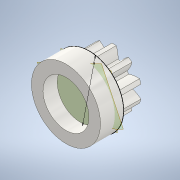
# Autodesk Inventor part: Spur Gear2
Saved by Autodesk Inventor 2022 (Build 260153070, 153G)
## iProperties
CustomPartVersion: 1
Created: 2021-10-29
Part Number: Spur Gear2
Material: Steel
Document SubType Name: Modeling
Designer: a laptop
Categories: <?xml version="1.0" encoding="UTF-16"?> <MemberInstance><Categories><FamilyTemplate><FamilyTemplateParameter ValueType="xs:double" Id="1" ObjectReferenceKey="da_z" ObjectType="kUserParameterObject"/><FamilyTemplateParameter ValueType="xs:double" Id="2" ObjectReferenceKey="da_b" ObjectType="kUserParameterObject"/><FamilyTemplateParameter ValueType="xs:double" Id="3" ObjectReferenceKey="da_beta" ObjectType="kUserParameterObject"/><FamilyTemplateParameter ValueType="xs:double" Id="4" ObjectReferenceKey="da_da" ObjectType="kUserParameterObject"/><FamilyTemplateParameter ValueType="xs:double" Id="5" ObjectReferenceKey="da_aw" ObjectType="kUserParameterObject"/><FamilyTemplateParameter ValueType="xs:string" Id="6" ObjectReferenceKey="EAIAABAAAACIAQAAAAAAAIAAAAAAAAAA" ObjectType="83910656" SubObjectId="SurfaceGeometry"/></FamilyTemplate><ParamToTemplateMap><ParamToTemplate CategoryParameter="//CategoryParameter[@InternalName='046C89C9-8512-4d59-83FE-43B91F4F132A']" TemplateParameter="1"/><ParamToTemplate CategoryParameter="//CategoryParameter[@InternalName='2552DF32-E462-4b46-AEBF-C6C7768E72AC']" TemplateParameter="2"/><ParamToTemplate CategoryParameter="//CategoryParameter[@InternalName='C9EE641D-15FC-4fae-A226-E94C4372FDD7']" TemplateParameter="3"/><ParamToTemplate><ParamToTemplate CategoryParameter="//CategoryParameter[@InternalName='00B6519A-459B-49c7-AD84-2E56D39A5744']" ConstantValue="0.000000"/></ParamToTemplate><ParamToTemplate><ParamToTemplate CategoryParameter="//CategoryParameter[@InternalName='04B31F0E-C7A6-4894-AA32-9629BEFACF47']" ConstantValue="1.000000"/></ParamToTemplate><ParamToTemplate><ParamToTemplate CategoryParameter="//CategoryParameter[@InternalName='43CBEC2E-7847-49e7-A936-2F7889FCB2D9']" ConstantValue="0.250000"/></ParamToTemplate><ParamToTemplate><ParamToTemplate CategoryParameter="//CategoryParameter[@InternalName='B1EFC894-105D-4ebd-86BF-FA20ED196853']" ConstantValue="0.302500"/></ParamToTemplate><ParamToTemplate><ParamToTemplate CategoryParameter="//CategoryParameter[@InternalName='51175063-3D10-4879-93E8-6246FE8B403D']" ConstantValue="2060000000.000000"/></ParamToTemplate><ParamToTemplate><ParamToTemplate CategoryParameter="//CategoryParameter[@InternalName='A3A52E27-4454-46a9-B0BD-C932399B70AF']" ConstantValue="0.300000"/></ParamToTemplate><ParamToTemplate><ParamToTemplate CategoryParameter="//CategoryParameter[@InternalName='91B76062-C214-41d9-B1B9-14D2AB99603D']" ConstantValue="0.060000"/></ParamToTemplate><ParamToTemplate><ParamToTemplate CategoryParameter="//CategoryParameter[@InternalName='374E806E-8B8A-4dda-A9AA-1039D6500AD2']" ConstantValue="16.666667"/></ParamToTemplate><ParamToTemplate><ParamToTemplate CategoryParameter="//CategoryParameter[@InternalName='2D373A89-B862-43d6-8D0B-0CBF12AB9F6C']" ConstantValue="0.349066"/></ParamToTemplate><ParamToTemplate CategoryParameter="//CategoryParameter[@InternalName='37777632-D6A2-4fac-9D53-DB8ACD95C989']" TemplateParameter="4"/><ParamToTemplate CategoryParameter="//CategoryParameter[@InternalName='FD1017F1-B727-4f7e-9707-0F86F1FF9423']" TemplateParameter="5"/><ParamToTemplate><ParamToTemplate CategoryParameter="//CategoryParameter[@InternalName='9E1B4470-B2D3-4ff1-B813-535BB4CDF51A']" ConstantValue="3520000.000000"/></ParamToTemplate><ParamToTemplate><ParamToTemplate CategoryParameter="//CategoryParameter[@InternalName='F8452263-BFF6-458c-9FB1-07C4B99E95CD']" ConstantValue="11400000.000000"/></ParamToTemplate><ParamToTemplate><ParamToTemplate CategoryParameter="//CategoryParameter[@InternalName='3E3BB259-FD49-497f-8171-6EBC954A3479']" ConstantValue="2.000000"/></ParamToTemplate><ParamToTemplate CategoryParameter="//CategoryParameter[@InternalName='27C3BAF2-7550-4e4b-AE2C-0DB134B7D9B7']" TemplateParameter="6"/></ParamToTemplateMap><Category DisplayName="Gear" InternalName="DC85795E-93AB-48d5-8EEE-5A27447B64BD" Mnemonic="Gear"><CategoryParameter DisplayName="z" InternalName="046C89C9-8512-4d59-83FE-43B91F4F132A" Mnemonic="z"/><CategoryParameter DisplayName="b" InternalName="2552DF32-E462-4b46-AEBF-C6C7768E72AC" Mnemonic="b"/><CategoryParameter DisplayName="||b|" InternalName="C9EE641D-15FC-4fae-A226-E94C4372FDD7" Mnemonic="beta"/><CategoryParameter DisplayName="x" InternalName="00B6519A-459B-49c7-AD84-2E56D39A5744" Mnemonic="x"/><CategoryParameter DisplayName="a*" InternalName="04B31F0E-C7A6-4894-AA32-9629BEFACF47" Mnemonic="a"/><CategoryParameter DisplayName="c*" InternalName="43CBEC2E-7847-49e7-A936-2F7889FCB2D9" Mnemonic="c"/><CategoryParameter DisplayName="r|.f|*" InternalName="B1EFC894-105D-4ebd-86BF-FA20ED196853" Mnemonic="rf"/><CategoryParameter DisplayName="E" InternalName="51175063-3D10-4879-93E8-6246FE8B403D" Mnemonic="E"/><CategoryParameter DisplayName="||m|" InternalName="A3A52E27-4454-46a9-B0BD-C932399B70AF" Mnemonic="mi"/><Category DisplayName="SpurGear" InternalName="26C5A22E-A91E-4dfd-A3B3-23CCAFAE1764" Mnemonic="SpurGear"><CategoryParameter DisplayName="m" InternalName="91B76062-C214-41d9-B1B9-14D2AB99603D" Mnemonic="m"/><CategoryParameter DisplayName="P" InternalName="374E806E-8B8A-4dda-A9AA-1039D6500AD2" Mnemonic="PP"/><CategoryParameter DisplayName="||a|" InternalName="2D373A89-B862-43d6-8D0B-0CBF12AB9F6C" Mnemonic="alpha"/><CategoryParameter DisplayName="d|.a|" InternalName="37777632-D6A2-4fac-9D53-DB8ACD95C989" Mnemonic="da"/><CategoryParameter DisplayName="a|.w|" InternalName="FD1017F1-B727-4f7e-9707-0F86F1FF9423" Mnemonic="aw"/><CategoryParameter DisplayName="||s||.Flim|" InternalName="9E1B4470-B2D3-4ff1-B813-535BB4CDF51A" Mnemonic="sFlim"/><CategoryParameter DisplayName="||s||.Hlim|" InternalName="F8452263-BFF6-458c-9FB1-07C4B99E95CD" Mnemonic="sHlim"/><CategoryParameter DisplayName="type" InternalName="3E3BB259-FD49-497f-8171-6EBC954A3479" Mnemonic="type"/><CategoryParameter DisplayName="PitchDiameter" InternalName="27C3BAF2-7550-4e4b-AE2C-0DB134B7D9B7" Mnemonic="IDS_PITCHDIAM"/></Category></Category></Categories></MemberInstance>
Density: 1 g/cm^3
Appearance: Steel
Author: a laptop
Autodesk Inventor part; units mm, degrees
ref_plane "YZ Plane" through (0, 0, 0) normal (1, 0, 0) x (0, 1, 0)
ref_plane "XZ Plane" through (0, 0, 0) normal (0, 1, 0) x (-1, 0, 0)
ref_plane "XY Plane" through (0, 0, 0) normal (0, 0, 1) x (1, 0, 0)
sketch "Sketch1" plane through (0, 0, 0) normal (0, 0, 1) x (1, 0, 0)
  circle A0 centre (0, 0) radius 3.6
  dimension "d0" = 7.2
  constraints: 1 centre point
  measures "d0" diameter of A0
extrude "Extrusion1" add sketch "Sketch1" along normal mid plane 3
ref_plane "Work Plane2" through (0, 0, 0) normal (0, 0, 1) x (1, 0, 0)
sketch "Sketch2" plane through (0, 0, -1.5) normal (0, 0, -1) x (-1, 0, 0)
  circle A0 centre (0, 0) radius 3.6 projected
  circle A1 centre (0, 0) radius 3
  dimension "d3" = 6
  constraints: 1 centre point, 1 coincident
  measures "d3" diameter of A1
surface extrude "Pitch Diameter" sketch "Sketch2" against normal through all shown no curves A1
ref_plane "Work Plane8" through (0, 0, 0) normal (0.9510565, 0.309017, 0) x (0, 0, 1)
ref_plane "Work Plane9" through (0, 0, 0) normal (1, 0, 0) x (0, 1, 0)
spur gear teeth "Spur Gear" teeth 10 pitch diameter 6 tip diameter 7.2 root diameter 4.5 face width 3 start plane through (0, 0, -1.5) normal (0, 0, -1) x (-1, 0, 0)
ref_plane "Work Plane12" through (0, 0, 2.9078) normal (0, 0, -1) x (-0.9035673, -0.4284463, 0)
ref_plane "Work Plane14" through (0, 0, 1.7684) normal (0, 0, -1) x (0.1129829, -0.9935969, 0)
sketch "Sketch6" plane through (0, 0, 1.7684) normal (0, 0, -1) x (0.1129829, -0.9935969, 0)
  arc A0 (-3.5978, -0.1248) -> (-3.534, -0.6861) centre (0, 0) ccw projected
  arc A1 (-0.9513, -2.039) -> (-0.9931, -3.4603) centre (2.2346, -2.8438) ccw projected
  arc A2 (-3.2624, 1.5221) -> (-2.1627, 0.6207) centre (-0.6786, 3.5524) ccw projected
  arc A3 (-3.5978, -0.1248) -> (-3.534, -0.6861) centre (0, 0) ccw projected
  arc A4 (-2.1627, 0.6207) -> (-2.2332, 0.2747) centre (0, 0) ccw projected
  arc A5 (-3.534, -0.6861) -> (-2.1145, -0.7691) centre (-2.6371, 2.4751) ccw projected
  arc A6 (-1.9681, -1.0904) -> (-2.8373, -2.2158) centre (0.1363, -3.6141) ccw projected
  arc A7 (-2.2332, 0.2747) -> (-3.5978, -0.1248) centre (-2.0141, -3.004) ccw projected
  arc A8 (-3.5978, -0.1248) -> (-3.534, -0.6861) centre (0, 0) ccw projected
  arc A9 (-2.1145, -0.7691) -> (-1.9681, -1.0904) centre (0, 0) ccw projected
  arc A10 (-1.2586, -1.8651) -> (-0.9513, -2.039) centre (0, 0) ccw projected
  arc A11 (-2.8373, -2.2158) -> (-2.4558, -2.6323) centre (0, 0) ccw projected
  arc A12 (-0.9931, -3.4603) -> (-0.4395, -3.5731) centre (0, 0) ccw projected
  arc A13 (-0.4395, -3.5731) -> (0.078, -2.2486) centre (-3.1689, -1.7432) ccw projected
  arc A14 (0.078, -2.2486) -> (0.4288, -2.2088) centre (0, 0) ccw projected
  arc A15 (0.4288, -2.2088) -> (1.2305, -3.3832) centre (3.4793, -0.9872) ccw projected
  arc A16 (1.2305, -3.3832) -> (1.7446, -3.149) centre (0, 0) ccw projected
  arc A17 (1.7446, -3.149) -> (1.3848, -1.7733) centre (-1.539, -3.2729) ccw projected
  arc A18 (1.3848, -1.7733) -> (1.6452, -1.5349) centre (0, 0) ccw projected
  arc A19 (1.6452, -1.5349) -> (2.9841, -2.0138) centre (3.3951, 1.2464) ccw projected
  arc A20 (2.9841, -2.0138) -> (3.2624, -1.5221) centre (0, 0) ccw projected
  arc A21 (3.2624, -1.5221) -> (2.1627, -0.6207) centre (0.6786, -3.5524) ccw projected
  arc A22 (2.1627, -0.6207) -> (2.2332, -0.2747) centre (0, 0) ccw projected
  arc A23 (2.2332, -0.2747) -> (3.5978, 0.1248) centre (2.0141, 3.004) ccw projected
  arc A24 (3.534, 0.6861) -> (2.1145, 0.7691) centre (2.6371, -2.4751) ccw projected
  arc A25 (-3.5978, -0.1248) -> (-3.534, -0.6861) centre (0, 0) ccw projected
  arc A26 (2.1145, 0.7691) -> (1.9681, 1.0904) centre (0, 0) ccw projected
  arc A27 (1.9681, 1.0904) -> (2.8373, 2.2158) centre (-0.1363, 3.6141) ccw projected
  arc A28 (-3.5978, -0.1248) -> (-3.534, -0.6861) centre (0, 0) ccw projected
  arc A29 (2.4558, 2.6323) -> (1.2586, 1.8651) centre (3.5883, -0.4523) ccw projected
  arc A30 (1.2586, 1.8651) -> (0.9513, 2.039) centre (0, 0) ccw projected
  arc A31 (0.9513, 2.039) -> (0.9931, 3.4603) centre (-2.2346, 2.8438) ccw projected
  arc A32 (0.4395, 3.5731) -> (-0.078, 2.2486) centre (3.1689, 1.7432) ccw projected
  arc A33 (-3.5978, -0.1248) -> (-3.534, -0.6861) centre (0, 0) ccw projected
  arc A34 (-3.5978, -0.1248) -> (-3.534, -0.6861) centre (0, 0) ccw projected
  arc A35 (-1.7446, 3.149) -> (-1.3848, 1.7733) centre (1.539, 3.2729) ccw projected
  arc A36 (-1.6452, 1.5349) -> (-2.9841, 2.0138) centre (-3.3951, -1.2464) ccw projected
  arc A37 (-3.5978, -0.1248) -> (-3.534, -0.6861) centre (0, 0) ccw projected
  arc A38 (-3.5978, -0.1248) -> (-3.534, -0.6861) centre (0, 0) ccw projected
  arc A39 (-1.3848, 1.7733) -> (-1.6452, 1.5349) centre (0, 0) ccw projected
  arc A40 (-0.078, 2.2486) -> (-0.4288, 2.2088) centre (0, 0) ccw projected
  arc A41 (-3.5978, -0.1248) -> (-3.534, -0.6861) centre (0, 0) ccw projected
  arc A42 (-3.5978, -0.1248) -> (-3.534, -0.6861) centre (0, 0) ccw projected
  arc A43 (-3.5978, -0.1248) -> (-3.534, -0.6861) centre (0, 0) ccw projected
  arc A44 (-3.5978, -0.1248) -> (-3.534, -0.6861) centre (0, 0) ccw projected
  circle A45 centre (0, 0) radius 4.5
  arc A46 (-2.4558, -2.6323) -> (-1.2586, -1.8651) centre (-3.5883, 0.4523) ccw projected
  arc A47 (0.9931, 3.4603) -> (0.4395, 3.5731) centre (0, 0) ccw projected
  arc A48 (2.8373, 2.2158) -> (2.4558, 2.6323) centre (0, 0) ccw projected
  arc A49 (3.5978, 0.1248) -> (3.534, 0.6861) centre (0, 0) ccw projected
  arc A50 (-0.4288, 2.2088) -> (-1.2305, 3.3832) centre (-3.4793, 0.9872) ccw projected
  arc A51 (-1.2305, 3.3832) -> (-1.7446, 3.149) centre (0, 0) ccw projected
  point P0 (0, 0)
  dimension "d60" = 9
  constraints: 1 centre point, 1 coincident
  measures "d60" diameter of A45
extrude "Extrusion4" add sketch "Sketch6" against normal blind 3
sketch "Sketch5" plane through (0, 0, 2.9078) normal (0, 0, -1) x (-0.9035673, -0.4284463, 0)
  circle A0 centre (0, 0) radius 3
  point P0 (0, 0)
  dimension "d53" = 6
  constraints: 1 centre point, 1 coincident
  measures "d53" diameter of A0
extrude "Extrusion3" cut sketch "Sketch5" against normal blind 20
sketch "Sketch7" plane through (0, 0, 1.5) normal (0, 0, 1) x (1, 0, 0)
  arc A0 (2.338, -2.7375) -> (1.7109, -1.4613) centre (-0.8549, -3.5142) ccw projected
  arc A1 (1.881, -3.0695) -> (2.338, -2.7375) centre (0, 0) ccw projected
  arc A2 (0.861, -2.0787) -> (1.881, -3.0695) centre (3.6064, -0.2729) ccw projected
  arc A3 (0.2825, -3.5889) -> (0.5253, -2.1878) centre (-2.7572, -2.3406) ccw projected
  arc A4 (-0.2825, -3.5889) -> (0.2825, -3.5889) centre (0, 0) ccw projected
  arc A5 (-0.5253, -2.1878) -> (-0.2825, -3.5889) centre (2.7572, -2.3406) ccw projected
  arc A6 (-0.861, -2.0787) -> (-0.5253, -2.1878) centre (0, 0) ccw projected
  arc A7 (-1.881, -3.0695) -> (-0.861, -2.0787) centre (-3.6064, -0.2729) ccw projected
  arc A8 (-1.7109, -1.4613) -> (-2.338, -2.7375) centre (0.8549, -3.5142) ccw projected
  arc A9 (-2.338, -2.7375) -> (-1.881, -3.0695) centre (0, 0) ccw projected
  arc A10 (-3.326, -1.3777) -> (-1.9184, -1.1756) centre (-3.078, 1.899) ccw projected
  arc A11 (-3.5005, -0.8404) -> (-3.326, -1.3777) centre (0, 0) ccw projected
  arc A12 (-2.2431, -0.1765) -> (-3.5005, -0.8404) centre (-1.374, -3.3455) ccw projected
  arc A13 (-3.5005, 0.8404) -> (-2.2431, 0.1765) centre (-1.374, 3.3455) ccw projected
  arc A14 (-2.2431, 0.1765) -> (-2.2431, -0.1765) centre (0, 0) ccw projected
  arc A15 (-3.326, 1.3777) -> (-3.5005, 0.8404) centre (0, 0) ccw projected
  arc A16 (-1.9184, 1.1756) -> (-3.326, 1.3777) centre (-3.078, -1.899) ccw projected
  arc A17 (-1.7109, 1.4613) -> (-1.9184, 1.1756) centre (0, 0) ccw projected
  arc A18 (-2.338, 2.7375) -> (-1.7109, 1.4613) centre (0.8549, 3.5142) ccw projected
  arc A19 (-0.861, 2.0787) -> (-1.881, 3.0695) centre (-3.6064, 0.2729) ccw projected
  arc A20 (-1.881, 3.0695) -> (-2.338, 2.7375) centre (0, 0) ccw projected
  arc A21 (-0.5253, 2.1878) -> (-0.861, 2.0787) centre (0, 0) ccw projected
  arc A22 (-0.2825, 3.5889) -> (-0.5253, 2.1878) centre (2.7572, 2.3406) ccw projected
  arc A23 (0.2825, 3.5889) -> (-0.2825, 3.5889) centre (0, 0) ccw projected
  arc A24 (0.5253, 2.1878) -> (0.2825, 3.5889) centre (-2.7572, 2.3406) ccw projected
  arc A25 (0.861, 2.0787) -> (0.5253, 2.1878) centre (0, 0) ccw projected
  arc A26 (1.881, 3.0695) -> (0.861, 2.0787) centre (3.6064, 0.2729) ccw projected
  arc A27 (2.338, 2.7375) -> (1.881, 3.0695) centre (0, 0) ccw projected
  arc A28 (1.7109, 1.4613) -> (2.338, 2.7375) centre (-0.8549, 3.5142) ccw projected
  arc A29 (1.9184, 1.1756) -> (1.7109, 1.4613) centre (0, 0) ccw projected
  arc A30 (3.326, 1.3777) -> (1.9184, 1.1756) centre (3.078, -1.899) ccw projected
  arc A31 (3.5005, 0.8404) -> (3.326, 1.3777) centre (0, 0) ccw projected
  arc A32 (2.2431, 0.1765) -> (3.5005, 0.8404) centre (1.374, 3.3455) ccw projected
  arc A33 (2.2431, -0.1765) -> (2.2431, 0.1765) centre (0, 0) ccw projected
  arc A34 (3.5005, -0.8404) -> (2.2431, -0.1765) centre (1.374, -3.3455) ccw projected
  arc A35 (3.326, -1.3777) -> (3.5005, -0.8404) centre (0, 0) ccw projected
  arc A36 (1.9184, -1.1756) -> (3.326, -1.3777) centre (3.078, 1.899) ccw projected
  arc A37 (1.7109, -1.4613) -> (1.9184, -1.1756) centre (0, 0) ccw projected
  arc A38 (0.5253, -2.1878) -> (0.861, -2.0787) centre (0, 0) ccw projected
  arc A39 (-1.9184, -1.1756) -> (-1.7109, -1.4613) centre (0, 0) ccw projected
extrude "Extrusion5" add sketch "Sketch7" along normal up to next
equation "\"d0\" = da_da"
equation "\"d1\" = da_b"
equation "\"d3\" = da_d"
equation "\"d16\" = da_aw"
equation "\"d43\" = da_aw"
equation "\"d46\" = da_aw"
equation "\"da_da\" = 7.2"
equation "\"da_b\" = 3"
equation "\"da_d\" = 6"
equation "\"da_aw\" = 21"
body "Solid1"
body "Srf1"
